Autodesk Fusion 360 part; units mm, degrees
note: some values were not read from the file. Set by a fixed rule: which face or edge a step refers to.
(part 4 of 5)
sketch "Sketch107" plane through (0, 0, 125) normal (0, 0, 1) x (-1, 0, 0)
  circle A0 centre (-11, -175) radius 3.5
  circle A1 centre (-199, -175) radius 3.5
  circle A2 centre (-11, -35) radius 3.5
  circle A3 centre (-199, -35) radius 3.5
  circle A4 centre (-199, -140) radius 2
  circle A5 centre (-11, -140) radius 2
  circle A6 centre (-199, -70) radius 2
  circle A7 centre (-11, -70) radius 2
  line L0 (-185.1631, -104.8) -> (-188.6631, -104.8)
  line L1 (-188.6631, -104.8) -> (-188.6631, -99.2)
  line L2 (-188.6631, -99.2) -> (-185.1631, -99.2)
  line L3 (-185.1631, -99.2) -> (-185.1631, -104.8)
  line L4 (-21.3369, -104.8) -> (-24.8369, -104.8)
  line L5 (-24.8369, -104.8) -> (-24.8369, -99.2)
  line L6 (-24.8369, -99.2) -> (-21.3369, -99.2)
  line L7 (-21.3369, -99.2) -> (-21.3369, -104.8)
  line L8 (-137, -11.1307) -> (-137, 0)
  line L9 (-137, 0) -> (-180, 0)
  arc A8 (-180, 0) -> (-210, -30) centre (-180, -30) ccw
  line L10 (-210, -30) -> (-210, -180)
  arc A9 (-210, -180) -> (-180, -210) centre (-180, -180) ccw
  line L11 (-180, -210) -> (-30, -210)
  arc A10 (-30, -210) -> (0, -180) centre (-30, -180) ccw
  line L12 (0, -180) -> (0, -30)
  arc A11 (0, -30) -> (-30, 0) centre (-30, -30) ccw
  line L13 (-30, 0) -> (-98.0333, 0)
  line L14 (-98.0333, 0) -> (-98.0333, -11)
  line L15 (-98.0333, -11) -> (-75, -11)
  spline S0 degree 3 poles (-75, -11) (-73.6669, -11) (-72.3215, -11.1868) (-70.7827, -11.5209) (-69.7039, -11.7551) (-68.5449, -12.0678) (-67.3101, -12.4666) (-63.5716, -13.6741) (-59.3264, -15.5672) (-54.921, -17.8316) (-52.6617, -18.993) (-50.3688, -20.252) (-48.1137, -21.5656) (-43.134, -24.4661) (-38.3659, -27.5905) (-34.4467, -30.5403) (-31.6285, -32.6614) (-29.2725, -34.6734) (-27.4088, -36.5974) (-26.9392, -37.0821) (-26.4696, -37.5669) (-26, -38.0516) knots 0 0 0 0 0.068385 0.068385 0.068385 0.116327 0.116327 0.116327 0.262353 0.262353 0.262353 0.337245 0.337245 0.337245 0.502934 0.502934 0.502934 0.621914 0.621914 0.621914 0.656812 0.656812 0.656812 0.656812
  line L16 (-26, -38.0516) -> (-26, -155.5)
  line L17 (-26, -155.5) -> (-13, -155.5)
  line L18 (-13, -160.5) -> (-18, -160.5)
  line L19 (-18, -160.5) -> (-18, -186.5)
  line L20 (-18, -186.5) -> (-25, -186.5)
  line L21 (-25, -186.5) -> (-25, -160.5)
  line L22 (-25, -160.5) -> (-26, -160.5)
  line L23 (-26, -160.5) -> (-26, -183)
  line L24 (-26, -183) -> (-101.02, -183)
  ellipse E0 centre (-105, -188.2858) end of major axis (-105, -180.5592) minor radius 5.4567 (-108.98, -183) -> (-101.02, -183) ccw
  line L25 (-184, -183) -> (-184, -160.5)
  line L26 (-184, -160.5) -> (-185, -160.5)
  line L27 (-185, -160.5) -> (-185, -186.5)
  line L28 (-185, -186.5) -> (-192, -186.5)
  line L29 (-192, -186.5) -> (-192, -160.5)
  line L30 (-192, -160.5) -> (-197, -160.5)
  line L31 (-197, -155.5) -> (-184, -155.5)
  line L32 (-184, -155.5) -> (-184, -38.0508)
  spline S1 degree 3 poles (-184, -38.0508) (-183.53, -37.5659) (-183.0599, -37.0811) (-182.5899, -36.5963) (-180.4883, -34.4285) (-177.7611, -32.1455) (-174.4691, -29.7357) (-169.3238, -25.9693) (-162.8741, -21.9475) (-156.519, -18.5779) (-152.2041, -16.29) (-147.9761, -14.3309) (-144.2124, -12.9853) (-141.9329, -12.1703) (-139.8769, -11.6068) (-138.0391, -11.287) (-137.6862, -11.2256) (-137.3408, -11.1732) (-137, -11.1307) knots -0.65681 -0.65681 -0.65681 -0.65681 -0.621923 -0.621923 -0.621923 -0.48793 -0.48793 -0.48793 -0.278155 -0.278155 -0.278155 -0.135918 -0.135918 -0.135918 -0.050335 -0.050335 -0.050335 -0.033901 -0.033901 -0.033901 -0.033901
  circle A12 centre (-11, -140) radius 2
  circle A13 centre (-11, -70) radius 2
  line L33 (-116.6351, 18) -> (-180, -5)
  arc A14 (-180, -5) -> (-205, -30) centre (-180, -30) ccw
  line L34 (-205, -30) -> (-205, -50)
  line L35 (-205, -50) -> (-190, -50)
  line L36 (-190, -50) -> (-190, -150)
  line L37 (-190, -150) -> (-205, -150)
  line L38 (-205, -150) -> (-205, -180)
  arc A15 (-205, -180) -> (-180, -205) centre (-180, -180) ccw
  line L39 (-180, -205) -> (-30, -205)
  arc A16 (-30, -205) -> (-5, -180) centre (-30, -180) ccw
  line L40 (-5, -180) -> (-5, -150)
  line L41 (-5, -150) -> (-20, -150)
  line L42 (-20, -150) -> (-20, -50)
  line L43 (-20, -50) -> (-5, -50)
  line L44 (-5, -50) -> (-5, -30)
  arc A17 (-5, -30) -> (-30, -5) centre (-30, -30) ccw
  line L45 (-30, -5) -> (-93.3667, 18)
  arc A18 (0, -30) -> (-30, 0) centre (-30, -30) ccw
  line L46 (0, -30) -> (0, -180)
  arc A19 (-30, -210) -> (0, -180) centre (-30, -180) ccw
  line L47 (-30, -210) -> (-180, -210)
  arc A20 (-210, -180) -> (-180, -210) centre (-180, -180) ccw
  line L48 (-210, -180) -> (-210, -30)
  arc A21 (-180, 0) -> (-210, -30) centre (-180, -30) ccw
  circle A22 centre (-199, -140) radius 2
  circle A23 centre (-199, -70) radius 2
  line L49 (-185, -195) -> (-195, -185)
  line L50 (-195, -185) -> (-200, -190)
  line L51 (-200, -190) -> (-190, -200)
  line L52 (-190, -200) -> (-185, -195)
  line L53 (-198, -165) -> (-200, -165)
  line L54 (-200, -165) -> (-200, -157.5)
  line L55 (-200, -157.5) -> (-198, -157.5)
  line L56 (-198, -157.5) -> (-198, -165)
  line L57 (-202, -165) -> (-204, -165)
  line L58 (-204, -165) -> (-204, -157.5)
  line L59 (-204, -157.5) -> (-202, -157.5)
  line L60 (-202, -157.5) -> (-202, -165)
  line L61 (-186.4142, -196.4142) -> (-196.4142, -186.4142)
  line L62 (-188.5858, -198.5858) -> (-198.5858, -188.5858)
  line L63 (-190, -152) -> (-190, -150.5)
  line L64 (-189.5, -140.5) -> (-188, -140.5)
  line L65 (-188, -140.5) -> (-188, -135.5)
  line L66 (-188, -135.5) -> (-189.5, -135.5)
  line L67 (-189.5, -135.5) -> (-189.5, -140.5)
  line L68 (-186, -140.5) -> (-184, -140.5)
  line L69 (-184, -140.5) -> (-184, -135.5)
  line L70 (-184, -135.5) -> (-186, -135.5)
  line L71 (-186, -135.5) -> (-186, -140.5)
  line L72 (-189.75, -50) -> (-187.75, -50)
  line L73 (-187.75, -50) -> (-187.75, -60)
  line L74 (-187.75, -60) -> (-189.75, -60)
  line L75 (-189.75, -60) -> (-189.75, -50)
  line L76 (-186, -50) -> (-184, -50)
  line L77 (-184, -50) -> (-184, -55)
  line L78 (-184, -55) -> (-186, -55)
  line L79 (-186, -55) -> (-186, -50)
  line L80 (-197, -160.5) -> (-198, -160.5)
  line L81 (-197, -155.5) -> (-198, -155.5)
  line L82 (-108.98, -183) -> (-184, -183)
  line L83 (-105, -191.1402) -> (-105, -26.9364)
  line L84 (-20.25, -50) -> (-22.25, -50)
  line L85 (-22.25, -50) -> (-22.25, -60)
  line L86 (-20.25, -60) -> (-20.25, -50)
  line L87 (-22.25, -60) -> (-20.25, -60)
  line L88 (-26, -135.5) -> (-24, -135.5)
  line L89 (-20.5, -140.5) -> (-22, -140.5)
  line L90 (-24, -140.5) -> (-26, -140.5)
  line L91 (-22, -140.5) -> (-22, -135.5)
  line L92 (-24, -135.5) -> (-24, -140.5)
  line L93 (-20.5, -135.5) -> (-20.5, -140.5)
  line L94 (-26, -140.5) -> (-26, -135.5)
  line L95 (-22, -135.5) -> (-20.5, -135.5)
  line L96 (-6, -165) -> (-6, -157.5)
  line L97 (-12, -157.5) -> (-12, -165)
  line L98 (-13, -160.5) -> (-13, -155.5)
  line L99 (-13, -155.5) -> (-12, -155.5)
  line L100 (-12, -165) -> (-10, -165)
  line L101 (-8, -157.5) -> (-8, -165)
  line L102 (-8, -165) -> (-6, -165)
  line L103 (-10, -157.5) -> (-12, -157.5)
  line L104 (-6, -157.5) -> (-8, -157.5)
  line L105 (-10, -165) -> (-10, -157.5)
  line L106 (-13, -160.5) -> (-12, -160.5)
  line L107 (-23.5858, -196.4142) -> (-13.5858, -186.4142)
  line L108 (-10, -190) -> (-20, -200)
  line L109 (-25, -195) -> (-15, -185)
  line L110 (-20, -200) -> (-25, -195)
  line L111 (-15, -185) -> (-10, -190)
  line L112 (-21.4142, -198.5858) -> (-11.4142, -188.5858)
  line L113 (-13, -155.5) -> (-13, -160.5)
  line L114 (-197, -160.5) -> (-197, -155.5)
  line L115 (-93.3667, 18) -> (-116.6351, 18)
  line L116 (-180, 0) -> (-116.6351, 23)
  line L117 (-116.6351, 23) -> (-93.3667, 23)
  line L118 (-93.3667, 23) -> (-30, 0)
  circle A24 centre (-11, -70) radius 2
  circle A25 centre (-199, -70) radius 2
  circle A26 centre (-11, -140) radius 2
  circle A27 centre (-199, -140) radius 2
  circle A28 centre (-199, -35) radius 3.5
  circle A29 centre (-11, -35) radius 3.5
  circle A30 centre (-199, -175) radius 3.5
  circle A31 centre (-11, -175) radius 3.5
  line L119 (-185.1631, -104.8) -> (-188.6631, -104.8)
  line L120 (-188.6631, -104.8) -> (-188.6631, -99.2)
  line L121 (-188.6631, -99.2) -> (-185.1631, -99.2)
  line L122 (-185.1631, -99.2) -> (-185.1631, -104.8)
  line L123 (-21.3369, -104.8) -> (-24.8369, -104.8)
  line L124 (-24.8369, -104.8) -> (-24.8369, -99.2)
  line L125 (-24.8369, -99.2) -> (-21.3369, -99.2)
  line L126 (-21.3369, -99.2) -> (-21.3369, -104.8)
  line L127 (-137, -11.1307) -> (-137, 0)
  line L128 (-137, 0) -> (-180, 0)
  arc A32 (-180, 0) -> (-210, -30) centre (-180, -30) ccw
  line L129 (-210, -30) -> (-210, -180)
  arc A33 (-210, -180) -> (-180, -210) centre (-180, -180) ccw
  line L130 (-180, -210) -> (-30, -210)
  arc A34 (-30, -210) -> (0, -180) centre (-30, -180) ccw
  line L131 (0, -180) -> (0, -30)
  arc A35 (0, -30) -> (-30, 0) centre (-30, -30) ccw
  line L132 (-30, 0) -> (-98.0333, 0)
  line L133 (-98.0333, 0) -> (-98.0333, -11)
  line L134 (-98.0333, -11) -> (-75, -11)
  spline S2 degree 3 poles (-75, -11) (-73.6669, -11) (-72.3215, -11.1868) (-70.7827, -11.5209) (-69.7039, -11.7551) (-68.5449, -12.0678) (-67.3101, -12.4666) (-63.5716, -13.6741) (-59.3264, -15.5672) (-54.921, -17.8316) (-52.6617, -18.993) (-50.3688, -20.252) (-48.1137, -21.5656) (-43.134, -24.4661) (-38.3659, -27.5905) (-34.4467, -30.5403) (-31.6285, -32.6614) (-29.2725, -34.6734) (-27.4088, -36.5974) (-26.9392, -37.0821) (-26.4696, -37.5669) (-26, -38.0516) knots 0 0 0 0 0.068385 0.068385 0.068385 0.116327 0.116327 0.116327 0.262353 0.262353 0.262353 0.337245 0.337245 0.337245 0.502934 0.502934 0.502934 0.621914 0.621914 0.621914 0.656812 0.656812 0.656812 0.656812
  line L135 (-26, -38.0516) -> (-26, -157.5)
  line L136 (-26, -157.5) -> (-12.5, -157.5)
  line L137 (-18, -160.5) -> (-18, -186.5)
  line L138 (-18, -186.5) -> (-25, -186.5)
  line L139 (-25, -186.5) -> (-25, -160.5)
  line L140 (-26, -183) -> (-101.02, -183)
  ellipse E1 centre (-105, -188.2858) end of major axis (-105, -180.5592) minor radius 5.4567 (-108.98, -183) -> (-101.02, -183) ccw
  line L141 (-108.98, -183) -> (-184, -183)
  line L142 (-184, -183) -> (-184, -160.5)
  line L143 (-185, -160.5) -> (-185, -186.5)
  line L144 (-185, -186.5) -> (-192, -186.5)
  line L145 (-192, -186.5) -> (-192, -160.5)
  line L146 (-197.5, -157.5) -> (-184, -157.5)
  line L147 (-184, -157.5) -> (-184, -38.0508)
  spline S3 degree 3 poles (-184, -38.0508) (-183.53, -37.5659) (-183.0599, -37.0811) (-182.5899, -36.5963) (-180.4883, -34.4285) (-177.7611, -32.1455) (-174.4691, -29.7357) (-169.3238, -25.9693) (-162.8741, -21.9475) (-156.519, -18.5779) (-152.2041, -16.29) (-147.9761, -14.3309) (-144.2124, -12.9853) (-141.9329, -12.1703) (-139.8769, -11.6068) (-138.0391, -11.287) (-137.6862, -11.2256) (-137.3408, -11.1732) (-137, -11.1307) knots -0.65681 -0.65681 -0.65681 -0.65681 -0.621923 -0.621923 -0.621923 -0.48793 -0.48793 -0.48793 -0.278155 -0.278155 -0.278155 -0.135918 -0.135918 -0.135918 -0.050335 -0.050335 -0.050335 -0.033901 -0.033901 -0.033901 -0.033901
  line L148 (-197.5, -155.5) -> (-184, -155.5)
  line L149 (-12.5, -157.5) -> (-12.5, -162.5)
  line L150 (-197.5, -162.5) -> (-197.5, -157.5)
  line L151 (-184, -157.5) -> (-197.5, -157.5)
  line L152 (-196.5, -162.5) -> (-197.5, -162.5)
  line L153 (-13.5, -160.5) -> (-18, -160.5)
  line L154 (-26, -160.5) -> (-26, -183)
  line L155 (-184, -160.5) -> (-185, -160.5)
  line L156 (-12.5, -162.5) -> (-13.5, -162.5)
  line L157 (-13.5, -162.5) -> (-13.5, -160.5)
  line L158 (-25, -160.5) -> (-26, -160.5)
  line L159 (-192, -160.5) -> (-196.5, -160.5)
  line L160 (-196.5, -160.5) -> (-196.5, -162.5)
  point P0 (-20, -150.5)
  point P1 (-20, -150)
  point P2 (-18, -160.5)
  point P3 (-25, -186.5)
  point P4 (-18, -186.5)
  dimension "d957" = 2
  dimension "d958" = 2
  dimension "d960" = 1.5
  dimension "d961" = 5
  dimension "d962" = 2
  dimension "d963" = 10
  dimension "d964" = 0.25
  dimension "d967" = 2
  dimension "d968" = 2
  dimension "d1052" = 15
  constraint perpendicular L49 L50
  constraint perpendicular L50 L51
  constraint perpendicular L49 L52
  constraint horizontal L53
  constraint vertical L54
  constraint horizontal L55
  constraint vertical L56
  constraint horizontal L57
  constraint vertical L58
  constraint horizontal L59
  constraint vertical L60
  constraint coincident L52 L61.start
  constraint coincident L50 L61.end
  constraint perpendicular L50 L61
  constraint coincident L52 L62.start
  constraint coincident L50 L62.end
  constraint parallel L61 L62
  constraint vertical L63
  constraint collinear L36 L63
  constraint horizontal L64
  constraint vertical L65
  constraint horizontal L66
  constraint vertical L67
  constraint horizontal L68
  constraint vertical L69
  constraint horizontal L70
  constraint vertical L71
  constraint horizontal L72
  constraint vertical L73
  constraint horizontal L74
  constraint vertical L75
  constraint horizontal L76
  constraint vertical L77
  constraint horizontal L78
  constraint vertical L79
  constraint collinear L32 L77
  constraint coincident L30.end L80.start
  constraint coincident L56 L80.end
  constraint perpendicular L56 L80
  constraint coincident L31.start L81.start
  constraint coincident L56 L81.end
  constraint perpendicular L56 L81
  constraint symmetric L72.start L83 L84.start
  constraint symmetric L72.end L83 L84.end
  constraint symmetric L73.end L83 L85.end
  constraint symmetric L74.end L83 L86.start
  constraint symmetric L29.end L83 P2
  constraint symmetric L30.end L83 L18.start
  constraint symmetric L31.start L83 L17.end
  constraint symmetric L36.end L83 P1
  constraint symmetric L53.start L83 L97.end
  constraint symmetric L53.end L83 L100.end
  constraint symmetric L54.end L83 L103.start
  constraint symmetric L55.end L83 L97.start
  constraint symmetric L57.start L83 L101.end
  constraint symmetric L57.end L83 L96.start
  constraint symmetric L58.end L83 L96.end
  constraint symmetric L59.end L83 L101.start
  constraint symmetric L63.end L83 P0
  constraint symmetric L64.start L83 L89.start
  constraint symmetric L64.end L83 L89.end
  constraint symmetric L65.end L83 L91.end
  constraint symmetric L66.end L83 L93.start
  constraint symmetric L68.start L83 L90.start
  constraint symmetric L68.end L83 L90.end
  constraint symmetric L69.end L83 L88.start
  constraint symmetric L70.end L83 L88.end
  constraint symmetric L80.end L83 L106.end
  constraint symmetric L81.end L83 L99.end
  constraint symmetric L27.end L83 P3
  constraint symmetric L28.end L83 P4
  constraint symmetric L49.start L83 L109.start
  constraint symmetric L49.end L83 L109.end
  constraint symmetric L50.end L83 L108.start
  constraint symmetric L51.end L83 L108.end
  constraint symmetric L61.start L83 L107.start
  constraint symmetric L61.end L83 L107.end
  constraint symmetric L62.start L83 L112.start
  constraint symmetric L62.end L83 L112.end
  constraint collinear L64 L68
  constraint collinear L66 L70
  constraint collinear L55 L59
  constraint collinear L55 L151
  measures "d957" distance of L49 L61
  measures "d958" distance of L51 L62
  measures "d960" distance of L64.start L64.end
  measures "d961" distance of L64.start L66.end
  measures "d962" distance of L72.start L72.end
  measures "d963" distance of L72.start L74.end
  measures "d964" distance of L36 L75
  measures "d967" distance of L77.end L78.end
  measures "d968" distance of L68.start L68.end
  measures "d1052" distance of L68 L148
extrude "Extrude62" cut sketch "Sketch95" against normal blind 5 contours L7 L8 L9 L10 L11 L12 L20 L23 | L21 L70 L71 L72 L73 L74 bodies 5 in component "inner_adapter"
extrude "Extrude61" add sketch "Sketch107" along normal blind 10 separate body contours L32 L68 L69 L70 L71 L147 | L16 L88 L90 L92 L94 L135 | L49 L50 L52 L61 | L50 L51 L52 L62 | L53 L54 L55 L56 | L57 L58 L59 L60 | L64 L65 L66 L67 | L72 L73 L74 L75 | L84 L85 L86 L87 | L89 L91 L93 L95 | L96 L101 L102 L104 | L97 L100 L103 L105 | L107 L109 L110 L111 | L108 L110 L111 L112 makes body 14 at (189.7475, 193.0809, 128.3333) makes body 15 at (20.25, 56.6667, 128.3333) makes body 16 at (8, 160, 128.3333) makes body 17 at (200, 162.5, 128.3333) makes body 18 at (187.75, 53.3333, 128.3333) makes body 19 at (204, 162.5, 128.3333) makes body 20 at (10, 162.5, 128.3333) makes body 21 at (24, 137.1667, 128.3333) makes body 22 at (21.6667, 191.6667, 128.3333) makes body 23 at (189.5, 137.1667, 128.3333) makes body 24 at (184, 138.8333, 128.3333) makes body 25 at (22, 138.8333, 128.3333) makes body 26 at (196.6667, 193.3333, 128.3333) makes body 27 at (13.3333, 193.3333, 128.3333) in component "inner_adapter"
sketch "Sketch116" plane through (0, 0, 135) normal (0, 0, 1) x (-1, 0, 0)
  line L0 (-189.75, -60) -> (-187.75, -60)
  line L1 (-187.75, -60) -> (-187.75, -50)
  line L2 (-187.75, -50) -> (-189.75, -50)
  line L3 (-189.75, -50) -> (-189.75, -60)
  line L4 (-189.75, -50) -> (-185, -50)
  line L5 (-185, -50) -> (-185, -60)
  line L6 (-185, -60) -> (-189.75, -60)
  line L7 (-189.75, -60) -> (-189.75, -50)
  line L8 (-189.5, -135.5) -> (-189.5, -140.5)
  line L9 (-189.5, -140.5) -> (-188, -140.5)
  line L10 (-188, -140.5) -> (-188, -135.5)
  line L11 (-188, -135.5) -> (-189.5, -135.5)
  line L12 (-189.5, -135.5) -> (-186.5, -135.5)
  line L13 (-186.5, -135.5) -> (-186.5, -140.5)
  line L14 (-186.5, -140.5) -> (-189.5, -140.5)
  line L15 (-189.5, -140.5) -> (-189.5, -135.5)
  line L16 (-202, -157.5) -> (-204, -157.5)
  line L17 (-204, -157.5) -> (-204, -165)
  line L18 (-204, -165) -> (-202, -165)
  line L19 (-202, -165) -> (-202, -157.5)
  line L20 (-188.5858, -198.5858) -> (-198.5858, -188.5858)
  line L21 (-198.5858, -188.5858) -> (-200, -190)
  line L22 (-200, -190) -> (-190, -200)
  line L23 (-190, -200) -> (-188.5858, -198.5858)
  line L24 (-204, -157.5) -> (-200.5, -157.5)
  line L25 (-200.5, -157.5) -> (-200.5, -164.9406)
  line L26 (-200.5, -164.9406) -> (-204, -164.9406)
  line L27 (-204, -164.9406) -> (-204, -157.5)
  line L28 (-200, -190) -> (-196.818, -186.818)
  line L29 (-190, -200) -> (-186.818, -196.818)
  line L30 (-186.818, -196.818) -> (-196.818, -186.818)
  line L31 (-105, -191.1402) -> (-105, -26.9364)
  line L32 (-20.25, -60) -> (-22.25, -60)
  line L33 (-20.25, -50) -> (-20.25, -60)
  line L34 (-25, -50) -> (-25, -60)
  line L35 (-20.25, -50) -> (-25, -50)
  line L36 (-25, -60) -> (-20.25, -60)
  line L37 (-20.25, -60) -> (-20.25, -50)
  line L38 (-22.25, -60) -> (-22.25, -50)
  line L39 (-22.25, -50) -> (-20.25, -50)
  line L40 (-8, -165) -> (-8, -157.5)
  line L41 (-20.5, -140.5) -> (-22, -140.5)
  line L42 (-6, -157.5) -> (-9.5, -157.5)
  line L43 (-20.5, -135.5) -> (-23.5, -135.5)
  line L44 (-20.5, -135.5) -> (-20.5, -140.5)
  line L45 (-9.5, -164.9406) -> (-6, -164.9406)
  line L46 (-10, -190) -> (-13.182, -186.818)
  line L47 (-21.4142, -198.5858) -> (-11.4142, -188.5858)
  line L48 (-11.4142, -188.5858) -> (-10, -190)
  line L49 (-23.182, -196.818) -> (-13.182, -186.818)
  line L50 (-20, -200) -> (-21.4142, -198.5858)
  line L51 (-20, -200) -> (-23.182, -196.818)
  line L52 (-10, -190) -> (-20, -200)
  line L53 (-6, -164.9406) -> (-6, -157.5)
  line L54 (-9.5, -157.5) -> (-9.5, -164.9406)
  line L55 (-23.5, -135.5) -> (-23.5, -140.5)
  line L56 (-6, -157.5) -> (-6, -165)
  line L57 (-22, -135.5) -> (-20.5, -135.5)
  line L58 (-20.5, -140.5) -> (-20.5, -135.5)
  line L59 (-22, -140.5) -> (-22, -135.5)
  line L60 (-8, -157.5) -> (-6, -157.5)
  line L61 (-6, -165) -> (-8, -165)
  line L62 (-23.5, -140.5) -> (-20.5, -140.5)
  dimension "d1056" = 3
  dimension "d1057" = 3.5
  dimension "d1058" = 4.5
  dimension "d1059" = 4.5
  constraint horizontal L4
  constraint vertical L5
  constraint horizontal L6
  constraint vertical L7
  constraint coincident L2.end L3.start
  constraint horizontal L12
  constraint vertical L13
  constraint horizontal L14
  constraint vertical L15
  constraint coincident L8.start L11.end
  constraint horizontal L24
  constraint vertical L25
  constraint horizontal L26
  constraint vertical L27
  constraint coincident L16.end L17.start
  constraint coincident L21.end L22.start
  constraint perpendicular L20 L28
  constraint coincident L22.end L23.start
  constraint perpendicular L22 L29
  constraint symmetric L0.start L31 L32.start
  constraint symmetric L0.end L31 L32.end
  constraint symmetric L1.end L31 L38.end
  constraint symmetric L2.end L31 L33.start
  constraint symmetric L4.end L31 L34.start
  constraint symmetric L5.end L31 L34.end
  constraint symmetric L8.start L31 L43.start
  constraint symmetric L8.end L31 L41.start
  constraint symmetric L9.end L31 L41.end
  constraint symmetric L10.end L31 L57.start
  constraint symmetric L12.end L31 L43.end
  constraint symmetric L13.end L31 L55.end
  constraint symmetric L16.start L31 L40.end
  constraint symmetric L16.end L31 L42.start
  constraint symmetric L17.end L31 L56.end
  constraint symmetric L18.end L31 L40.start
  constraint symmetric L20.start L31 L47.start
  constraint symmetric L20.end L31 L47.end
  constraint symmetric L21.end L31 L46.start
  constraint symmetric L22.end L31 L50.start
  constraint symmetric L24.end L31 L42.end
  constraint symmetric L25.end L31 L45.start
  constraint symmetric L26.end L31 L45.end
  constraint symmetric L28.end L31 L46.end
  constraint symmetric L29.end L31 L49.start
  measures "d1056" distance of L8.start L12.end
  measures "d1057" distance of L16.end L24.end
  measures "d1058" distance of L21.end L28.end
  measures "d1059" distance of L22.end L29.end
extrude "Extrude67" add sketch "Sketch116" along normal blind 4 bodies 25 27 18 19 23 26 16 15 in component "inner_adapter"
sketch "Sketch117" plane through (0, 50, 0) normal (0, -1, 0) x (1, 0, 0)
  line L0 (187.75, 125) -> (189.75, 125)
  line L1 (189.75, 125) -> (189.75, 139)
  line L2 (189.75, 139) -> (185, 139)
  line L3 (185, 139) -> (185, 135)
  line L4 (185, 135) -> (187.75, 135)
  line L5 (187.75, 135) -> (187.75, 125)
  line L6 (187.75, 135) -> (185, 139)
  constraint coincident L4.end L5.start
  constraint coincident L2.end L3.start
extrude "Extrude68" cut sketch "Sketch117" against normal blind 10 contours L3 L4 L6 bodies 18 in component "inner_adapter"
sketch "Sketch118" plane through (0, 135.5, 0) normal (0, -1, 0) x (1, 0, 0)
  line L0 (188, 125) -> (189.5, 125)
  line L1 (189.5, 125) -> (189.5, 139)
  line L2 (189.5, 139) -> (186.5, 139)
  line L3 (186.5, 139) -> (186.5, 135)
  line L4 (186.5, 135) -> (188, 135)
  line L5 (188, 135) -> (188, 125)
  line L6 (188, 135) -> (186.5, 139)
  constraint coincident L4.end L5.start
  constraint coincident L2.end L3.start
extrude "Extrude69" cut sketch "Sketch118" against normal blind 5 contours L3 L4 L6 bodies 23 in component "inner_adapter"
sketch "Sketch119" plane through (0, 157.5, 0) normal (0, -1, 0) x (1, 0, 0)
  line L0 (202, 125) -> (204, 125)
  line L1 (204, 125) -> (204, 139)
  line L2 (204, 139) -> (200.5, 139)
  line L3 (200.5, 139) -> (200.5, 135)
  line L4 (200.5, 135) -> (202, 135)
  line L5 (202, 135) -> (202, 125)
  line L6 (202, 135) -> (200.5, 139)
  constraint coincident L4.end L5.start
  constraint coincident L2.end L3.start
extrude "Extrude70" cut sketch "Sketch119" against normal blind 7.5 contours L3 L4 L6 bodies 19 in component "inner_adapter"
sketch "Sketch120" plane through (5, -5, 0) normal (0.707107, -0.707107, 0) x (0.707107, 0.707107, 0)
  line L0 (273.7716, 125) -> (275.7716, 125)
  line L1 (275.7716, 125) -> (275.7716, 139)
  line L2 (275.7716, 139) -> (271.2716, 139)
  line L3 (271.2716, 139) -> (271.2716, 135)
  line L4 (271.2716, 135) -> (273.7716, 135)
  line L5 (273.7716, 135) -> (273.7716, 125)
  line L6 (273.7716, 135) -> (271.2716, 139)
  constraint coincident L4.end L5.start
  constraint coincident L2.end L3.start
extrude "Extrude71" cut sketch "Sketch120" against normal blind 15 contours L3 L4 L6 bodies 26 in component "inner_adapter"
extrude "Extrude72" add 6 faces at (192.6095, 189.2761, 135) (198.6667, 162.5, 135) (185.3333, 137.1667, 135) (25.3333, 137.1667, 135) (11.3333, 160, 135) (21.1953, 192.1381, 135) along direction (0, 0, 1) blind 4 on bodies 14 17 20 21 22 24 bodies 14 5 25 27 17 18 19 22 20 23 26 16 15 21 24 in component "inner_adapter"
sketch "Sketch121" plane through (0, 50, 0) normal (0, -1, 0) x (1, 0, 0)
  line L0 (20.25, 125) -> (22.25, 125)
  line L1 (22.25, 125) -> (22.25, 135)
  line L2 (22.25, 135) -> (25, 135)
  line L3 (25, 135) -> (25, 139)
  line L4 (25, 139) -> (20.25, 139)
  line L5 (20.25, 139) -> (20.25, 125)
  line L6 (22.25, 135) -> (25, 139)
  constraint coincident L1.end L2.start
  constraint coincident L3.end L4.start
extrude "Extrude73" cut sketch "Sketch121" against normal blind 10 contours L2 L3 L6 bodies 15 in component "inner_adapter"
sketch "Sketch122" plane through (0, 135.5, 0) normal (0, -1, 0) x (1, 0, 0)
  line L0 (20.5, 125) -> (22, 125)
  line L1 (22, 125) -> (22, 135)
  line L2 (22, 135) -> (23.5, 135)
  line L3 (23.5, 135) -> (23.5, 139)
  line L4 (23.5, 139) -> (20.5, 139)
  line L5 (20.5, 139) -> (20.5, 125)
  line L6 (22, 135) -> (23.5, 139)
  constraint coincident L1.end L2.start
  constraint coincident L3.end L4.start
extrude "Extrude74" cut sketch "Sketch122" against normal blind 5 contours L2 L3 L6 bodies 25 in component "inner_adapter"
sketch "Sketch123" plane through (0, 157.5, 0) normal (0, -1, 0) x (1, 0, 0)
  line L0 (6, 125) -> (8, 125)
  line L1 (8, 125) -> (8, 135)
  line L2 (8, 135) -> (9.5, 135)
  line L3 (9.5, 135) -> (9.5, 139)
  line L4 (9.5, 139) -> (6, 139)
  line L5 (6, 139) -> (6, 125)
  line L6 (8, 135) -> (9.5, 139)
  constraint coincident L1.end L2.start
  constraint coincident L3.end L4.start
extrude "Extrude75" cut sketch "Sketch123" against normal blind 10 contours L2 L3 L6 bodies 16 in component "inner_adapter"
sketch "Sketch124" plane through (100, 100, 0) normal (-0.707107, -0.707107, 0) x (0.707107, -0.707107, 0)
  line L0 (-127.2792, 125) -> (-125.2792, 125)
  line L1 (-125.2792, 125) -> (-125.2792, 135)
  line L2 (-125.2792, 135) -> (-122.7792, 135)
  line L3 (-122.7792, 135) -> (-122.7792, 139)
  line L4 (-122.7792, 139) -> (-127.2792, 139)
  line L5 (-127.2792, 139) -> (-127.2792, 125)
  line L6 (-125.2792, 135) -> (-122.7792, 139)
  constraint coincident L1.end L2.start
  constraint coincident L3.end L4.start
extrude "Extrude76" cut sketch "Sketch124" against normal blind 15 contours L2 L3 L6 bodies 27 in component "inner_adapter"
extrude "Extrude64" cut 1 faces at (103.7762, 182.6498, 125) along direction (0, 0, 1) blind 5 on bodies 5 bodies 5 in component "inner_adapter"
sketch "Sketch110" plane through (0, 183, 0) normal (0, 1, 0) x (-1, 0, 0)
  circle A0 centre (-181.4998, 134.998) radius 1.9
  circle A1 centre (-28.5002, 134.998) radius 1.9
  line L0 (-108.98, 125) -> (-108.98, 130)
  line L1 (-108.98, 130) -> (-101.02, 130)
  line L2 (-101.02, 130) -> (-101.02, 125)
  line L3 (-101.02, 125) -> (-26, 125)
  line L4 (-26, 125) -> (-26, 205)
  line L5 (-26, 205) -> (-184, 205)
  line L6 (-184, 205) -> (-184, 125)
  line L7 (-184, 125) -> (-108.98, 125)
  circle A2 centre (-105, 170.0157) radius 5.25
  circle A3 centre (-45, 130) radius 2
  circle A4 centre (-45, 171) radius 2
  line L8 (-180, 125) -> (-30, 125)
  circle A5 centre (-132, 130) radius 2
  line L9 (-45, 130) -> (-132, 130)
  circle A6 centre (-132, 171) radius 2
  line L10 (-45, 171) -> (-132, 171)
  line L11 (-132, 171) -> (-132, 130)
  line L12 (-45, 130) -> (-45, 171)
  line L13 (-45, 130) -> (-40, 130)
  line L14 (-40, 130) -> (-40, 125)
  line L15 (-40, 125) -> (-45, 125)
  line L16 (-45, 125) -> (-45, 130)
  line L17 (-40, 125) -> (-50, 125)
  line L18 (-50, 125) -> (-50, 135)
  line L19 (-50, 135) -> (-40, 135)
  line L20 (-40, 135) -> (-40, 125)
  line L21 (-41.5, 125) -> (-48.5, 125)
  line L22 (-48.5, 125) -> (-48.5, 135)
  line L23 (-48.5, 135) -> (-41.5, 135)
  line L24 (-41.5, 135) -> (-41.5, 125)
  line L25 (-88.5, 130) -> (-88.5, 171)
  line L26 (-132, 150.5) -> (-45, 150.5)
  line L27 (-132, 125) -> (-132, 130)
  line L28 (-137, 130) -> (-137, 125)
  line L29 (-127, 125) -> (-127, 135)
  line L30 (-132, 130) -> (-137, 130)
  line L31 (-137, 125) -> (-127, 125)
  line L32 (-137, 135) -> (-137, 125)
  line L33 (-135.5, 135) -> (-135.5, 125)
  line L34 (-135.5, 125) -> (-128.5, 125)
  line L35 (-127, 135) -> (-137, 135)
  line L36 (-128.5, 125) -> (-128.5, 135)
  circle A7 centre (-132, 130) radius 2
  line L37 (-137, 125) -> (-132, 125)
  line L38 (-128.5, 135) -> (-135.5, 135)
  circle A8 centre (-132, 171) radius 2
  line L39 (-127, 176) -> (-127, 166)
  line L40 (-137, 176) -> (-127, 176)
  line L41 (-128.5, 176) -> (-128.5, 166)
  line L42 (-132, 176) -> (-132, 171)
  line L43 (-132, 171) -> (-137, 171)
  line L44 (-137, 176) -> (-132, 176)
  line L45 (-135.5, 176) -> (-128.5, 176)
  line L46 (-128.5, 166) -> (-135.5, 166)
  line L47 (-137, 166) -> (-137, 176)
  line L48 (-127, 166) -> (-137, 166)
  line L49 (-135.5, 166) -> (-135.5, 176)
  circle A9 centre (-132, 171) radius 2
  line L50 (-137, 171) -> (-137, 176)
  line L51 (-41.5, 176) -> (-48.5, 176)
  line L52 (-41.5, 166) -> (-41.5, 176)
  line L53 (-45, 171) -> (-40, 171)
  line L54 (-48.5, 166) -> (-41.5, 166)
  line L55 (-40, 166) -> (-40, 176)
  circle A10 centre (-45, 171) radius 2
  line L56 (-48.5, 176) -> (-48.5, 166)
  line L57 (-40, 176) -> (-50, 176)
  line L58 (-40, 171) -> (-40, 176)
  line L59 (-50, 166) -> (-40, 166)
  line L60 (-40, 176) -> (-45, 176)
  line L61 (-45, 176) -> (-45, 171)
  line L62 (-50, 176) -> (-50, 166)
  point P0 (-132, 171)
  dimension "d987" = 4
  dimension "d988" = 4
  dimension "d989" = 41
  dimension "d990" = 5
  dimension "d991" = 4
  dimension "d992" = 87
  dimension "d993" = 4
  dimension "d998" = 5
  dimension "d999" = 5
  dimension "d1000" = 10
  dimension "d1001" = 10
  dimension "d1002" = 7
  dimension "d1003" = 10
  dimension "d1004" = 1.5
  constraint coincident A3.centre L9.start
  constraint coincident A5.centre L9.end
  constraint parallel L8 L9
  constraint coincident A4.centre L10.start
  constraint coincident P0 A6.centre
  constraint parallel L9 L10
  constraint perpendicular L10 L12
  constraint parallel L11 L12
  constraint horizontal L13
  constraint vertical L14
  constraint horizontal L15
  constraint vertical L16
  constraint horizontal L17
  constraint vertical L18
  constraint horizontal L19
  constraint vertical L20
  constraint horizontal L21
  constraint vertical L22
  constraint horizontal L23
  constraint vertical L24
  constraint coincident L15 L21.start
  constraint midpoint L9 L25.start
  constraint midpoint L10 L25.end
  constraint midpoint L11 L26.start
  constraint midpoint L12 L26.end
  constraint symmetric A3 L25 A7
  constraint symmetric A3.centre L25 A5.centre
  constraint symmetric L13.end L25 L28.start
  constraint symmetric L14.end L25 L28.end
  constraint symmetric L15.end L25 L27.start
  constraint symmetric L17.end L25 L29.start
  constraint symmetric L18.end L25 L29.end
  constraint symmetric L19.end L25 L32.start
  constraint symmetric L21.start L25 L33.end
  constraint symmetric L21.end L25 L34.end
  constraint symmetric L22.end L25 L36.end
  constraint symmetric L23.end L25 L33.start
  constraint symmetric A5 L26 A9
  constraint symmetric A5.centre L26 P0
  constraint symmetric L26 A5.centre P0
  constraint symmetric L26 L28.start L43.end
  constraint symmetric L26 L28.end L40.start
  constraint symmetric L26 L27.start L42.start
  constraint symmetric L26 L34.end L41.start
  constraint symmetric L26 L29.end L39.end
  constraint symmetric L26 L33.start L46.end
  constraint symmetric L26 L29.start L39.start
  constraint symmetric L26 L33.end L45.start
  constraint symmetric L26 L36.end L41.end
  constraint symmetric L26 L32.start L47.start
  constraint symmetric L26 A7 A8
  constraint symmetric A3 L26 A10
  constraint symmetric A3.centre L26 A4.centre
  constraint symmetric L13.end L26 L53.end
  constraint symmetric L14.end L26 L55.end
  constraint symmetric L15.end L26 L60.end
  constraint symmetric L17.end L26 L57.end
  constraint symmetric L18.end L26 L59.start
  constraint symmetric L19.end L26 L55.start
  constraint symmetric L21.start L26 L51.start
  constraint symmetric L21.end L26 L51.end
  constraint symmetric L22.end L26 L54.start
  constraint symmetric L23.end L26 L52.start
  measures "d987" diameter of A3
  measures "d988" diameter of A4
  measures "d989" distance of A3.centre A4.centre
  measures "d990" distance of A3.centre L8
  measures "d991" diameter of A5
  measures "d992" horizontal distance of A3.centre A5.centre
  measures "d993" diameter of A6
  measures "d998" distance of A3.centre L13.end
  measures "d999" distance of A3.centre L15.end
  measures "d1000" distance of L14.end L17.end
  measures "d1001" distance of L14.end L19.end
  measures "d1002" distance of L21.start L21.end
  measures "d1003" distance of L21.start L23.end
  measures "d1004" distance of L18 L22
extrude "Extrude65" add sketch "Sketch110" along normal blind 8 contours L7 L8 L9 L29 L31 L36 | L9 L29 L35 L36 | L3 L8 L9 L17 L18 L22 | L9 L18 L19 L22 | L7 L8 L28 L30 L31 L32 L33 L37 | L30 L32 L33 L35 | L3 L8 L13 L14 L15 L17 L20 L24 | L10 L56 L57 L62 | L10 L56 L59 L62 | L13 L19 L20 L24 | L10 L39 L41 L48 | L43 L47 L48 L49 | L52 L53 L55 L59 | L10 L39 L40 L41 | L40 L43 L44 L47 L49 L50 | L52 L53 L55 L57 L58 L60 bodies 5 in component "inner_adapter"
extrude "Extrude66" add sketch "Sketch110" along normal blind 4.5 from surface at 3.5 contours L7 L8 A5 L9 L27 L31 L34 L36 A7 | A5 L9 L11 L35 L36 A7 L38 | L7 L8 A5 L27 L30 L31 L33 L34 A7 L37 | L3 A3 L8 L9 L16 L17 L21 L22 | L3 A3 L8 L13 L15 L16 L17 L21 L24 | A3 L9 L12 L19 L22 L23 | A5 L11 L30 L33 L35 A7 L38 | A6 L11 A8 L43 L46 L48 L49 A9 | A6 L10 L11 A8 L41 L46 L48 A9 | A3 L12 L13 L19 L23 L24 | A4 L10 L12 L54 A10 L56 L59 | A4 L12 L52 L53 L54 A10 L59 | A4 L10 L51 A10 L56 L57 L61 | A6 A8 L40 L42 L43 L44 L45 L49 A9 | A6 L10 A8 L40 L41 L42 L45 A9 | A4 L51 L52 L53 A10 L57 L60 L61 bodies 5 in component "inner_adapter"
sketch "Sketch111" plane through (0, 178, 0) normal (0, -1, 0) x (1, 0, 0)
  ellipse E0 centre (105, 105.4372) end of major axis (105, 112.1715) minor radius 4.7559
  line L0 (26, 1) -> (184, 1)
  line L1 (184, 1) -> (184, 115)
  line L2 (184, 115) -> (26, 115)
  line L3 (26, 115) -> (26, 1)
  ellipse E1 centre (105, 105.4372) end of major axis (105, 112.1715) minor radius 4.7559
  ellipse E2 centre (104.9954, 105.4372) end of major axis (105.0046, 114.1715) minor radius 6.7559
  line L4 (104.9954, 114.1715) -> (104.9954, 105.4372)
  line L5 (31, 115) -> (31, 25)
  line L6 (105, 105.4372) -> (179, 115)
  line L7 (105, 105.4372) -> (31, 115)
  point P0 (105, 98.7029)
  point P1 (179, 115)
  constraint coincident E2 L4.start
  constraint coincident E2.centre L4.end
  constraint parallel L4 L5
  constraint coincident E0.centre E1.centre
  constraint coincident P1 L6.end
  constraint coincident L5.start L7.end
extrude "Extrude25'" add sketch "Sketch111" along normal blind 7 contours E0 E1 E2 L4 L6 | E0 E1 E2 L4 L7 bodies 4 in component "Tunnel"
sketch "Sketch113" plane through (0, 0, 205) normal (0, 0, 1) x (-1, 0, 0)
  line L0 (-31, -171.5) -> (-26, -171.5)
  line L1 (-26, -171.5) -> (-26, -38.0516)
  spline S0 degree 3 poles (-26, -38.0516) (-26.4696, -37.5669) (-26.9392, -37.0821) (-27.4088, -36.5974) (-29.2725, -34.6734) (-31.6285, -32.6614) (-34.4467, -30.5403) (-38.3659, -27.5905) (-43.134, -24.4661) (-48.1137, -21.5656) (-50.3688, -20.252) (-52.6617, -18.993) (-54.921, -17.8316) (-59.3264, -15.5672) (-63.5716, -13.6741) (-67.3101, -12.4666) (-68.5449, -12.0678) (-69.7039, -11.7551) (-70.7827, -11.5209) (-72.3215, -11.1868) (-73.6669, -11) (-75, -11) knots -0.656812 -0.656812 -0.656812 -0.656812 -0.621914 -0.621914 -0.621914 -0.502934 -0.502934 -0.502934 -0.337245 -0.337245 -0.337245 -0.262353 -0.262353 -0.262353 -0.116327 -0.116327 -0.116327 -0.068385 -0.068385 -0.068385 0 0 0 0
  line L2 (-75, -11) -> (-135, -11)
  spline S1 degree 3 poles (-135, -11) (-135.3658, -11) (-135.7424, -11.0145) (-136.1336, -11.0437) (-136.7557, -11.0901) (-137.3844, -11.1731) (-138.0391, -11.287) (-139.8769, -11.6068) (-141.9329, -12.1703) (-144.2124, -12.9853) (-147.9761, -14.3309) (-152.2041, -16.29) (-156.519, -18.5779) (-162.8741, -21.9475) (-169.3238, -25.9693) (-174.4691, -29.7357) (-177.7611, -32.1455) (-180.4883, -34.4285) (-182.5899, -36.5963) (-183.0599, -37.0811) (-183.53, -37.5659) (-184, -38.0508) knots 0 0 0 0 0.019847 0.019847 0.019847 0.050335 0.050335 0.050335 0.135918 0.135918 0.135918 0.278155 0.278155 0.278155 0.48793 0.48793 0.48793 0.621923 0.621923 0.621923 0.65681 0.65681 0.65681 0.65681
  line L3 (-184, -38.0508) -> (-184, -171.5)
  line L4 (-184, -171.5) -> (-179, -171.5)
  line L5 (-179, -171.5) -> (-179, -40.0766)
  spline S2 degree 3 poles (-179, -40.0766) (-177.1947, -38.2144) (-174.6472, -36.0625) (-171.5158, -33.7703) (-166.6133, -30.1816) (-160.3099, -26.2473) (-154.1768, -22.9953) (-150.0182, -20.7903) (-145.9518, -18.9172) (-142.5291, -17.6934) (-139.736, -16.6948) (-137.3746, -16.1501) (-135.7618, -16.0299) (-135.486, -16.0093) (-135.2319, -16) (-135, -16) knots -0.621923 -0.621923 -0.621923 -0.621923 -0.48793 -0.48793 -0.48793 -0.278155 -0.278155 -0.278155 -0.135918 -0.135918 -0.135918 -0.019847 -0.019847 -0.019847 0 0 0 0
  line L6 (-135, -16) -> (-75, -16)
  spline S3 degree 3 poles (-75, -16) (-73.6407, -16) (-71.4915, -16.3704) (-68.8469, -17.2246) (-63.8244, -18.8468) (-57.0667, -22.1371) (-50.6302, -25.8861) (-45.8029, -28.6979) (-41.1682, -31.7394) (-37.4534, -34.5352) (-34.7859, -36.5429) (-32.601, -38.4237) (-31, -40.0763) knots 0 0 0 0 0.116327 0.116327 0.116327 0.337245 0.337245 0.337245 0.502934 0.502934 0.502934 0.621914 0.621914 0.621914 0.621914
  line L7 (-31, -40.0763) -> (-31, -171.5)
  line L8 (-26, -176.5) -> (-31, -176.5)
  line L9 (-31, -176.5) -> (-31, -178)
  line L10 (-31, -178) -> (-179, -178)
  line L11 (-179, -178) -> (-179, -176.5)
  line L12 (-179, -176.5) -> (-184, -176.5)
  line L13 (-184, -176.5) -> (-184, -183)
  line L14 (-184, -183) -> (-26, -183)
  line L15 (-26, -183) -> (-26, -176.5)
  line L16 (-185, -186.5) -> (-185, -160.5)
  line L17 (-185, -160.5) -> (-192, -160.5)
  line L18 (-192, -160.5) -> (-192, -186.5)
  line L19 (-192, -186.5) -> (-185, -186.5)
  line L20 (-25, -160.5) -> (-25, -186.5)
  line L21 (-25, -186.5) -> (-18, -186.5)
  line L22 (-18, -186.5) -> (-18, -160.5)
  line L23 (-18, -160.5) -> (-25, -160.5)
  line L24 (-184, -183) -> (-192, -183)
  line L25 (-192, -183) -> (-18, -183)
  line L26 (-18, -183) -> (-18, -186.5)
  line L27 (-18, -186.5) -> (-192, -186.5)
  line L28 (-192, -186.5) -> (-192, -183)
  line L29 (-192, -186.5) -> (-25.1398, -186.5)
  line L30 (-25.1398, -186.5) -> (-25.1398, -190.5)
  line L31 (-25.1398, -190.5) -> (-192, -190.5)
  line L32 (-192, -190.5) -> (-192, -186.5)
  line L33 (-184, -38.0508) -> (-192, -160.5)
  line L34 (-192, -160.5) -> (-194.2818, -195.4255)
  line L35 (-194.2818, -195.4255) -> (-198.2733, -195.1648)
  line L36 (-184, -38.0508) -> (-187.9915, -37.79)
  line L37 (-187.9915, -37.79) -> (-198.2733, -195.1648)
  line L38 (-192, -190.5) -> (-197.9685, -190.5)
  line L39 (-192, -186.5) -> (-193.6987, -186.5)
  spline S4 degree 3 poles (-135, -7) (-135.4719, -7) (-135.9483, -7.0188) (-136.4309, -7.0548) (-137.2067, -7.1126) (-137.9673, -7.2145) (-138.7248, -7.3463) (-140.848, -7.7157) (-143.1119, -8.3439) (-145.559, -9.2188) (-149.5874, -10.659) (-153.9573, -12.6921) (-158.3928, -15.0439) (-164.9221, -18.5059) (-171.496, -22.6022) (-176.8318, -26.5081) (-180.2458, -29.0071) (-183.1334, -31.4102) (-185.4619, -33.812) (-185.9319, -34.2969) (-186.4019, -34.7817) (-186.8719, -35.2665) knots 0 0 0 0 0.019847 0.019847 0.019847 0.050335 0.050335 0.050335 0.135918 0.135918 0.135918 0.278155 0.278155 0.278155 0.48793 0.48793 0.48793 0.621923 0.621923 0.621923 0.65681 0.65681 0.65681 0.65681
  spline S5 degree 3 poles (-23.127, -35.2685) (-23.5966, -34.7837) (-24.0662, -34.299) (-24.5358, -33.8142) (-26.6019, -31.6814) (-29.1079, -29.5522) (-32.0413, -27.3444) (-36.1216, -24.2734) (-41.0007, -21.0795) (-46.1004, -18.1091) (-48.414, -16.7616) (-50.7662, -15.4698) (-53.0924, -14.2741) (-57.6208, -11.9463) (-62.0214, -9.9713) (-66.0807, -8.6602) (-67.4303, -8.2243) (-68.7145, -7.8767) (-69.934, -7.612) (-71.6432, -7.2409) (-73.2933, -7) (-75, -7) knots -0.656812 -0.656812 -0.656812 -0.656812 -0.621914 -0.621914 -0.621914 -0.502934 -0.502934 -0.502934 -0.337245 -0.337245 -0.337245 -0.262353 -0.262353 -0.262353 -0.116327 -0.116327 -0.116327 -0.068385 -0.068385 -0.068385 0 0 0 0
  line L40 (-75, -7) -> (-135, -7)
  line L41 (-187.9915, -37.79) -> (-186.8719, -35.2665)
  line L42 (-26, -38.0516) -> (-18, -160.5)
  line L43 (-18, -160.5) -> (-15.7182, -195.4255)
  line L44 (-15.7182, -195.4255) -> (-11.7267, -195.1648)
  line L45 (-26, -38.0516) -> (-22.0085, -37.7909)
  line L46 (-22.0085, -37.7909) -> (-11.7267, -195.1648)
  line L47 (-23.127, -35.2685) -> (-22.0085, -37.7909)
  line L48 (-25.1398, -190.5) -> (-12.0315, -190.5)
  line L49 (-18, -186.5) -> (-16.3013, -186.5)
  line L50 (-185, -160.5) -> (-25, -160.5)
  dimension "d1020" = 4
  dimension "d1021" = 35
  dimension "d1022" = 4
  dimension "d1023" = 4
  dimension "d1024" = 4
  dimension "d1025" = 4
  dimension "d1026" = 35
  dimension "d1027" = 4
  dimension "d1028" = 4
  constraint coincident L13.end L14.start
  constraint coincident L18 L24.end
  constraint perpendicular L18 L24
  constraint horizontal L25
  constraint vertical L26
  constraint horizontal L27
  constraint vertical L28
  constraint coincident L21.end L22.start
  constraint horizontal L29
  constraint vertical L30
  constraint horizontal L31
  constraint vertical L32
  constraint coincident L18.end L19.start
  constraint coincident S1.end L3.start
  constraint coincident L17.end L18.start
  constraint parallel L33 L34
  constraint perpendicular L34 L35
  constraint perpendicular L33 L36
  constraint coincident L37 L38.end
  constraint perpendicular L32 L38
  constraint coincident L34 L39.end
  constraint perpendicular L28 L39
  constraint coincident L1.end S0.start
  constraint coincident L22.end L23.start
  constraint parallel L42 L43
  constraint perpendicular L43 L44
  constraint perpendicular L42 L45
  constraint coincident L46 L48.end
  constraint perpendicular L30 L48
  constraint coincident L43 L49.end
  constraint perpendicular L22 L49
  constraint coincident L16.end L17.start
  constraint coincident L20.start L23.end
  measures "d1020" distance of L18.end L31.end
  measures "d1021" distance of L17.end L34.end
  measures "d1022" distance of L34.end L35.end
  measures "d1023" distance of S1.end L36.end
  measures "d1026" distance of L22.end L43.end
  measures "d1027" distance of L43.end L44.end
  measures "d1028" distance of L1.end L45.end
extrude "Extrude61'" add sketch "Sketch113" against normal blind 6 separate body contours L1 L23 L42 L50 | L42 L43 L45 L46 L48 | S0 L2 S1 L36 S4 S5 L40 L41 L45 L47 | L3 L17 L33 L50 | L22 L26 L43 L49 | L14 L16 L20 L24 L25 L27 L29 | L33 L34 L36 L37 L38 | L21 L27 L30 L43 L48 L49 | L18 L28 L34 L39 | L19 L27 L29 L30 L31 L32 | L32 L34 L38 L39 makes body 28
sketch "Sketch114" plane through (0, 0, 205) normal (0, 0, 1) x (-1, 0, 0)
  line L0 (-192, -186.5) -> (-192, -160.5)
  line L1 (-192, -160.5) -> (-184, -160.5)
  line L2 (-184, -160.5) -> (-184, -38.0508)
  spline S0 degree 3 poles (-184, -38.0508) (-183.53, -37.5659) (-183.0599, -37.0811) (-182.5899, -36.5963) (-180.4883, -34.4285) (-177.7611, -32.1455) (-174.4691, -29.7357) (-169.3238, -25.9693) (-162.8741, -21.9475) (-156.519, -18.5779) (-152.2041, -16.29) (-147.9761, -14.3309) (-144.2124, -12.9853) (-141.9329, -12.1703) (-139.8769, -11.6068) (-138.0391, -11.287) (-137.3844, -11.1731) (-136.7557, -11.0901) (-136.1336, -11.0437) (-135.7424, -11.0145) (-135.3658, -11) (-135, -11) knots -0.65681 -0.65681 -0.65681 -0.65681 -0.621923 -0.621923 -0.621923 -0.48793 -0.48793 -0.48793 -0.278155 -0.278155 -0.278155 -0.135918 -0.135918 -0.135918 -0.050335 -0.050335 -0.050335 -0.019847 -0.019847 -0.019847 0 0 0 0
  line L3 (-135, -11) -> (-75, -11)
  spline S1 degree 3 poles (-75, -11) (-73.6669, -11) (-72.3215, -11.1868) (-70.7827, -11.5209) (-69.7039, -11.7551) (-68.5449, -12.0678) (-67.3101, -12.4666) (-63.5716, -13.6741) (-59.3264, -15.5672) (-54.921, -17.8316) (-52.6617, -18.993) (-50.3688, -20.252) (-48.1137, -21.5656) (-43.134, -24.4661) (-38.3659, -27.5905) (-34.4467, -30.5403) (-31.6285, -32.6614) (-29.2725, -34.6734) (-27.4088, -36.5974) (-26.9392, -37.0821) (-26.4696, -37.5669) (-26, -38.0516) knots 0 0 0 0 0.068385 0.068385 0.068385 0.116327 0.116327 0.116327 0.262353 0.262353 0.262353 0.337245 0.337245 0.337245 0.502934 0.502934 0.502934 0.621914 0.621914 0.621914 0.656812 0.656812 0.656812 0.656812
  line L4 (-26, -38.0516) -> (-26, -160.5)
  line L5 (-26, -160.5) -> (-18, -160.5)
  line L6 (-18, -160.5) -> (-18, -186.5)
  line L7 (-18, -186.5) -> (-25, -186.5)
  line L8 (-25, -186.5) -> (-25, -183)
  line L9 (-25, -183) -> (-185, -183)
  line L10 (-185, -183) -> (-185, -186.5)
  line L11 (-185, -186.5) -> (-192, -186.5)
  line L12 (-197.9685, -190.5) -> (-12.0315, -190.5)
  line L13 (-12.0315, -190.5) -> (-22.0085, -37.7909)
  line L14 (-22.0085, -37.7909) -> (-23.127, -35.2685)
  spline S2 degree 3 poles (-23.127, -35.2685) (-23.5966, -34.7837) (-24.0662, -34.299) (-24.5358, -33.8142) (-26.6019, -31.6814) (-29.1079, -29.5522) (-32.0413, -27.3444) (-36.1216, -24.2734) (-41.0007, -21.0795) (-46.1004, -18.1091) (-48.414, -16.7616) (-50.7662, -15.4698) (-53.0924, -14.2741) (-57.6208, -11.9463) (-62.0214, -9.9713) (-66.0807, -8.6602) (-67.4303, -8.2243) (-68.7145, -7.8767) (-69.934, -7.612) (-71.6432, -7.2409) (-73.2933, -7) (-75, -7) knots -0.656812 -0.656812 -0.656812 -0.656812 -0.621914 -0.621914 -0.621914 -0.502934 -0.502934 -0.502934 -0.337245 -0.337245 -0.337245 -0.262353 -0.262353 -0.262353 -0.116327 -0.116327 -0.116327 -0.068385 -0.068385 -0.068385 0 0 0 0
  line L15 (-75, -7) -> (-135, -7)
  spline S3 degree 3 poles (-135, -7) (-135.4719, -7) (-135.9483, -7.0188) (-136.4309, -7.0548) (-137.2067, -7.1126) (-137.9673, -7.2145) (-138.7248, -7.3463) (-140.848, -7.7157) (-143.1119, -8.3439) (-145.559, -9.2188) (-149.5874, -10.659) (-153.9573, -12.6921) (-158.3928, -15.0439) (-164.9221, -18.5059) (-171.496, -22.6022) (-176.8318, -26.5081) (-180.2458, -29.0071) (-183.1334, -31.4102) (-185.4619, -33.812) (-185.9319, -34.2969) (-186.4019, -34.7817) (-186.8719, -35.2665) knots 0 0 0 0 0.019847 0.019847 0.019847 0.050335 0.050335 0.050335 0.135918 0.135918 0.135918 0.278155 0.278155 0.278155 0.48793 0.48793 0.48793 0.621923 0.621923 0.621923 0.65681 0.65681 0.65681 0.65681
  line L16 (-186.8719, -35.2665) -> (-187.9915, -37.79)
  line L17 (-187.9915, -37.79) -> (-197.9685, -190.5)
  line L18 (-15.2339, -187.5) -> (-24.9673, -38.519)
  line L19 (-24.9673, -38.519) -> (-25.6531, -36.9725)
  spline S4 degree 3 poles (-25.6531, -36.9725) (-25.9989, -36.6155) (-26.3447, -36.2586) (-26.6905, -35.9016) (-28.6075, -33.9227) (-30.9965, -31.8855) (-33.8453, -29.7413) (-37.806, -26.7603) (-42.5997, -23.62) (-47.6104, -20.7015) (-49.8802, -19.3794) (-52.1877, -18.1123) (-54.4639, -16.9423) (-58.9032, -14.6603) (-63.1785, -12.7502) (-67.0027, -11.515) (-68.2666, -11.1068) (-69.4562, -10.7856) (-70.5706, -10.5437) (-72.1515, -10.2004) (-73.5756, -10) (-75, -10) knots -0.647613 -0.647613 -0.647613 -0.647613 -0.621914 -0.621914 -0.621914 -0.502934 -0.502934 -0.502934 -0.337245 -0.337245 -0.337245 -0.262353 -0.262353 -0.262353 -0.116327 -0.116327 -0.116327 -0.068385 -0.068385 -0.068385 0 0 0 0
  line L20 (-75, -10) -> (-135, -10)
  spline S5 degree 3 poles (-135, -10) (-135.3922, -10) (-135.794, -10.0156) (-136.2079, -10.0465) (-136.8683, -10.0957) (-137.5301, -10.1835) (-138.2105, -10.3018) (-140.1228, -10.6346) (-142.2256, -11.213) (-144.549, -12.0437) (-148.3823, -13.4142) (-152.6403, -15.3894) (-156.9875, -17.6944) (-163.3877, -21.088) (-169.865, -25.1262) (-175.0598, -28.9288) (-178.3847, -31.3627) (-181.1462, -33.6704) (-183.3079, -35.9002) (-183.654, -36.2572) (-184.0001, -36.6142) (-184.3463, -36.9713) knots 0 0 0 0 0.019847 0.019847 0.019847 0.050335 0.050335 0.050335 0.135918 0.135918 0.135918 0.278155 0.278155 0.278155 0.48793 0.48793 0.48793 0.621923 0.621923 0.621923 0.647614 0.647614 0.647614 0.647614
  line L21 (-184.3463, -36.9713) -> (-185.0327, -38.5184)
  line L22 (-185.0327, -38.5184) -> (-194.7661, -187.5)
  line L23 (-194.7661, -187.5) -> (-15.2339, -187.5)
  dimension "d1032" = -3
extrude "Extrude62'" cut sketch "Sketch114" against normal blind 2 from surface at -2 contours L12 L13 L14 S2 L15 S3 L16 L17 bodies 28
fillet "Fillet5" radius 5 2 edges at (197.9685, 190.5, 204) (197.9685, 190.5, 200) on bodies 28
fillet "Fillet6" radius 5 2 edges at (12.0315, 190.5, 200) (12.0315, 190.5, 204) on bodies 28
fillet "Fillet7" radius 5 1 edges at (15.2339, 187.5, 202) on bodies 28
fillet "Fillet8" radius 5 1 edges at (194.7661, 187.5, 202) on bodies 28